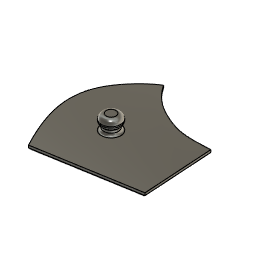
MaskPatternOutside v6 (Autodesk Fusion 360 design; units mm, degrees)
Autodesk Fusion 360 part; units mm, degrees
sketch "MaskV2" plane through (0, 0, 0) normal (0, 0, 1) x (1, 0, 0)
  spline S0 degree 5 poles (-34.2523, 95.3336) (-35.2526, 94.6891) (-37.2409, 93.3658) (-40.1864, 91.2783) (-44.0399, 88.2891) (-48.7276, 84.2113) (-53.2705, 79.8034) (-57.6389, 75.091) (-61.7831, 70.123) (-65.6362, 64.9683) (-69.1279, 59.6986) (-72.1952, 54.3745) (-74.7946, 49.0314) (-76.9151, 43.6626) (-78.5689, 38.2286) (-79.7757, 32.67) (-80.5515, 26.9191) (-80.8926, 20.9126) (-80.7756, 14.597) (-80.1673, 7.9268) (-79.031, 0.8656) (-77.3347, -6.6132) (-75.0591, -14.5257) (-72.1957, -22.8797) (-68.7429, -31.6769) (-64.7038, -40.9156) (-61.0077, -48.6568) (-57.9762, -54.6582) (-55.8403, -58.7457) (-54.7436, -60.8111) knots 0 0 0 0 0 0 0.04 0.08 0.12 0.16 0.2 0.24 0.28 0.32 0.36 0.4 0.44 0.48 0.52 0.56 0.6 0.64 0.68 0.72 0.76 0.8 0.84 0.88 0.92 0.96 1 1 1 1 1 1
  spline S1 degree 5 poles (69.5672, 53.3007) (67.8702, 53.1838) (64.548, 52.9705) (59.7802, 52.7121) (53.8562, 52.4908) (47.173, 52.4234) (41.1946, 52.571) (35.8717, 52.9412) (31.1095, 53.5427) (26.7456, 54.3847) (22.5564, 55.477) (18.3169, 56.8318) (13.8423, 58.4658) (9.0491, 60.4018) (3.9674, 62.668) (-1.3048, 65.2946) (-6.6318, 68.31) (-11.8738, 71.7374) (-16.9248, 75.5895) (-21.7215, 79.8688) (-26.2284, 84.5726) (-29.5909, 88.6705) (-31.975, 91.93) (-33.5034, 94.1853) (-34.2523, 95.3336) knots 0 0 0 0 0 0 0.05 0.1 0.15 0.2 0.25 0.3 0.35 0.4 0.45 0.5 0.55 0.6 0.65 0.7 0.75 0.8 0.85 0.9 0.95 1 1 1 1 1 1
  line L0 (37.7916, 52.8446) -> (43.3291, -44.1745)
  line L1 (-54.7436, -60.8111) -> (75.4385, -38.7276)
  line L2 (69.5672, 53.3007) -> (75.4385, -38.7276)
  circle A0 centre (-17.78, 10.16) radius 9.525
  circle A1 centre (-17.78, 10.16) radius 12.7
  line L3 (-33.8654, -49.2972) -> (47.6075, -34.9313) construction
  line L4 (47.6075, -34.9313) -> (44.2995, -16.1707) construction
  line L5 (44.2995, -16.1707) -> (-37.1734, -30.5366) construction
  line L6 (-37.1734, -30.5366) -> (-33.8654, -49.2972) construction
  dimension "d1" = 19.05
  dimension "d2" = 25.4
  constraint concentric A0 A1
  constraint perpendicular L3 L4
  constraint parallel L3 L5
  constraint parallel L4 L6
  measures "d1" diameter of A0
  measures "d2" diameter of A1
extrude "Extrude1" add sketch "MaskV2" against normal blind 6.35 contours S0 S1 L0 L1 | A0 | A1
extrude "Extrude2" add sketch "MaskV2" along normal blind 19.05 contours A0
extrude "Extrude3" add sketch "MaskV2" along normal blind 12.7 from surface at 6.35 contours A1
extrude "Extrude4" add sketch "MaskV2" against normal blind 6.35 contours S1 L0 L1 L2
fillet "Fillet1" radius 6.35 1 edges at (-29.6206, 5.5675, 19.05)
chamfer "Chamfer1" distance 3.175 angle 45 1 edges at (-29.6206, 5.5675, 6.35)
fillet "Fillet2" radius 3.81 1 edges at (-29.6206, 14.7525, 9.525)
chamfer "Chamfer2" distance 3.175 angle 45 6 edges at (-5.7072, -52.4928, -6.35) (-79.1174, 35.4295, -6.35) (2.2203, 63.5787, -6.35) (10.3475, -49.7693, -6.35) (72.5028, 7.2866, -6.35) (51.77, 52.4982, -6.35)
fillet "Fillet3" radius 3.175 1 edges at (-26.6604, 13.6044, 0)
